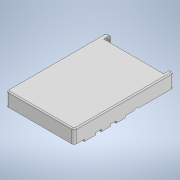
# Autodesk Inventor part: Pi 4 Case  - Upper Panel
Saved by Autodesk Inventor 2020 (Build 240168000, 168)
## iProperties
Created: 2021-01-01
Part Number: Pi 4 Case  - Upper Panel
Material: Generic
Document SubType Name: Modeling
Designer: frost
Density: 1 g/cm^3
Appearance: Default
Author: frost
Autodesk Inventor part; units mm, degrees
ref_plane "YZ Plane" through (0, 0, 0) normal (1, 0, 0) x (0, 1, 0)
ref_plane "XZ Plane" through (0, 0, 0) normal (0, 1, 0) x (-1, 0, 0)
ref_plane "XY Plane" through (0, 0, 0) normal (0, 0, 1) x (1, 0, 0)
sketch "Sketch1" plane through (0, 0, 0) normal (0, 1, 0) x (-1, 0, 0)
  line L0 (28, 44) -> (-28, 44)
  line L1 (-30, 42) -> (-30, -42)
  line L2 (-28, -44) -> (28, -44)
  line L3 (30, -42) -> (30, 42)
  line L4 (30, 44) -> (-30, -44) construction
  line L5 (-30, 44) -> (30, -44) construction
  line L6 (25, 42.5) -> (-25, 42.5)
  line L7 (-28, 39.5) -> (-28, -39.5)
  line L8 (-25, -42.5) -> (25, -42.5)
  line L9 (28, -39.5) -> (28, 39.5)
  line L10 (28, 42.5) -> (-28, -42.5) construction
  line L11 (-28, 42.5) -> (28, -42.5) construction
  arc A0 (25, -42.5) -> (28, -39.5) centre (25, -39.5) ccw
  arc A1 (-28, -39.5) -> (-25, -42.5) centre (-25, -39.5) ccw
  arc A2 (-25, 42.5) -> (-28, 39.5) centre (-25, 39.5) ccw
  arc A3 (28, 39.5) -> (25, 42.5) centre (25, 39.5) ccw
  arc A4 (-30, -42) -> (-28, -44) centre (-28, -42) ccw
  arc A5 (-28, 44) -> (-30, 42) centre (-28, 42) ccw
  arc A6 (28, -44) -> (30, -42) centre (28, -42) ccw
  arc A7 (30, 42) -> (28, 44) centre (28, 42) ccw
  point P0 (0, 0)
  dimension "d2" = 60
  dimension "d3" = 88
  dimension "d4" = 56
  dimension "d5" = 85
  dimension "d6" = 3
  dimension "d7" = 2
  constraints: 24 end point, 16 point on circle, 16 point on line, 16 tangent, 8 centre point, 6 equal radius, 4 midpoint, 4 parallel, 2 horizontal, 2 perpendicular
  measures "d2" distance of L4.end L5.end
  measures "d3" distance of L5.start L4.end
  measures "d4" distance of L11.end L10.end
  measures "d5" distance of L10.end L11.start
  measures "d6" radius of A0
  measures "d7" radius of A4
extrude "Extrusion1" add sketch "Sketch1" along normal blind 4 contours A7 L3 A6 L2 A4 L1 A5 L0 | A3 L9 A0 L8 A1 L7 A2 L6
extrude "Extrusion2" add sketch "Sketch1" against normal blind 8
sketch "Sketch2" plane through (28, 4, -44) normal (0, 0, -1) x (-1, 0, 0)
  line L0 (53, -12) -> (3, -12) projected
  line L1 (2, -1) -> (54, -1)
  line L2 (54, -1) -> (54, -12)
  line L3 (54, -12) -> (2, -12)
  line L4 (2, -12) -> (2, -1)
  line L5 (-2, -12) -> (-2, 0) projected
  line L6 (58, 0) -> (58, -12) projected
  point P0 (28, -4)
  dimension "d12" = 4
  dimension "d13" = 4
  dimension "d14" = 11
  constraints: 8 end point, 2 parallel, 1 horizontal, 1 perpendicular, 1 point on line
  measures "d12" distance between parallel lines of L5 L4
  measures "d13" distance between parallel lines of L6 L2
  measures "d14" distance of L1.end L2.end
extrude "Extrusion3" cut sketch "Sketch2" against normal blind 19
sketch "Sketch3" plane through (28, 4, -44) normal (0, 0, -1) x (-1, 0, 0)
  line L0 (2, -1) -> (54, -1) projected
  line L1 (54, -1) -> (38, -1)
  line L2 (38, -1) -> (38, -3.5)
  line L3 (38, -3.5) -> (54, -3.5)
  line L4 (54, -3.5) -> (54, -1)
  line L5 (0, 0) -> (56, 0) projected
  line L6 (2, -1) -> (54, -1)
  line L7 (54, -1) -> (54, 0)
  line L8 (54, 0) -> (2, 0)
  line L9 (2, 0) -> (2, -1)
  point P0 (28, -4)
  point P1 (38, -1)
  dimension "d17" = 16
  dimension "d18" = 2.5
  constraints: 16 end point, 4 parallel, 2 horizontal, 2 perpendicular, 1 point on line
  measures "d17" distance of L3.end L2.end
  measures "d18" distance of L2.end L1.end
extrude "Extrusion4" add sketch "Sketch3" against normal blind 21 contours L0 L4 L3 L2
extrude "Extrusion5" cut sketch "Sketch3" against normal blind 5
sketch "Sketch4" plane through (30, 4, 42) normal (1, 0, 0) x (0, 0, -1)
  line L0 (86, -12) -> (86, 0) projected
  line L1 (84, -12) -> (0, -12) projected
  circle A0 centre (53.5, -14.5) radius 3.5
  point P0 (42, -4)
  point P1 (51.0505, -12)
  point P2 (55.9495, -12)
  dimension "d27" = 2.5
  dimension "d28" = 32.5
  dimension "d29" = 7
  constraints: 1 centre point
  measures "d27" distance from line of L1 A0.centre
  measures "d28" distance from line of L0 A0.centre
  measures "d29" diameter of A0
extrude "Extrusion6" cut sketch "Sketch4" against normal blind 10 contours L1 A0 picked at (52.8865, -11.841)
sketch "Sketch5" plane through (30, 4, 42) normal (1, 0, 0) x (0, 0, -1)
  line L0 (-4.9094, -13.7) -> (89.7531, -13.7)
  line L1 (84, -12) -> (55.9495, -12) projected
  point P0 (42, -4)
  dimension "d32" = 1.7
  constraints: 2 end point, 1 horizontal
  measures "d32" distance between parallel lines of L1 L0
sketch "Sketch6" plane through (30, 4, 42) normal (1, 0, 0) x (0, 0, -1)
  line L0 (43, -10.0638) -> (43, -13.7)
  arc A0 (55.9495, -12) -> (51.0505, -12) centre (53.5, -14.5) ccw projected
  line L1 (35, -10.0638) -> (35, -13.7)
  line L2 (30, -13.7) -> (30, -10.0638)
  line L3 (22, -10.0638) -> (22, -13.7)
  line L4 (17, -10.0638) -> (17, -13.7)
  line L5 (7, -10.0638) -> (7, -13.7)
  line L6 (6.4702, -10.0638) -> (43, -10.0638)
  line L7 (-3.7275, -13.7) -> (104.8817, -13.7)
  line L8 (84, -12) -> (55.9495, -12) projected
  point P0 (42, -4)
  dimension "d33" = 10.5
  dimension "d34" = 8
  dimension "d35" = 5
  dimension "d36" = 8
  dimension "d37" = 5
  dimension "d38" = 10
  dimension "d39" = 1.7
  constraints: 16 end point, 11 point on line, 6 vertical, 2 horizontal
  measures "d33" distance from line of L0 A0.centre
  measures "d34" distance between parallel lines of L0 L1
  measures "d35" distance between parallel lines of L1 L2
  measures "d36" distance between parallel lines of L3 L2
  measures "d37" distance between parallel lines of L4 L3
  measures "d38" distance between parallel lines of L4 L5
  measures "d39" distance between parallel lines of L8 L7
extrude "Extrusion7" add sketch "Sketch6" against normal blind 2 contours L0 L7 L1 L6 | L2 L7 L3 L6 | L4 L7 L5 L6
fillet "Fillet1" radius 1 10 edges at (29.4142, 4, -43.4142) (27, 4, -44) (29.4142, 4, 43.4142) (0, 4, 44) (-29.4142, 4, 43.4142) (-30, 4, 0) (-29.4142, 4, -43.4142) (-27, 4, -44) (30, 4, 0) (0, 4, -39)
body "Solid1"
